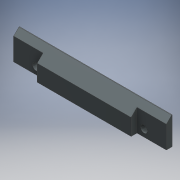
# Autodesk Inventor part: back_beam
Saved by Autodesk Inventor 2016 (Build 200138000, 138)
## iProperties
Created: 2017-01-15
Part Number: back_beam
Material: Generic
Document SubType Name: Modeling
Designer: hesaon
Density: 1 g/cm^3
Appearance: Default
Author: hesaon
Autodesk Inventor part; units mm, degrees
ref_plane "YZ Plane" through (0, 0, 0) normal (1, 0, 0) x (0, 1, 0)
ref_plane "XZ Plane" through (0, 0, 0) normal (0, 1, 0) x (-1, 0, 0)
ref_plane "XY Plane" through (0, 0, 0) normal (0, 0, 1) x (1, 0, 0)
sketch "Sketch1" plane through (0, 0, 0) normal (1, 0, 0) x (0, 1, 0)
  line L0 (0, 0) -> (0, -36)
  line L1 (0, -36) -> (-5, -36)
  line L2 (-5, -36) -> (-5, -5)
  line L3 (-5, -5) -> (0, 0)
  dimension "d1" = 5
  dimension "d2" = 45
  dimension "d5" = 31
  constraints: 8 end point, 2 perpendicular, 1 vertical
  measures "d1" distance of L0.end L1.end
  measures "d2" angle of L2 L3
  measures "d5" distance of L1.end L2.end
extrude "Extrusion1" add sketch "Sketch1" along normal blind 130
sketch "Sketch2" plane through (130, 0, 0) normal (1, 0, 0) x (0, 0, -1)
  line L0 (36, 0) -> (0, 0) projected
  line L1 (0, 0) -> (0.5, 0)
  line L2 (0.5, 0) -> (0.5, -0.5)
  line L3 (0, 0) -> (5, -5) projected
  line L4 (0, 0) -> (0.5, -0.5)
  dimension "d6" = 0.5
  constraints: 6 end point, 2 point on line, 1 collinear, 1 perpendicular
  measures "d6" distance of L0.end L1.end
extrude "Extrusion2" cut sketch "Sketch2" against normal through all
sketch "Sketch3" plane through (0, 0, -36) normal (0, 1, 0) x (1, 0, 0)
  circle A0 centre (19, -6) radius 3
  circle A1 centre (19, -18) radius 3
  line L0 (0, -35.5) -> (0, 0) projected
  line L1 (0, 0) -> (130, 0) projected
  circle A2 centre (111, -6) radius 3
  circle A3 centre (111, -18) radius 3
  line L2 (130, 0) -> (130, -35.5) projected
  point P0 (0, -36)
  dimension "d9" = 6
  dimension "d10" = 6
  dimension "d11" = 19
  dimension "d12" = 12
  dimension "d13" = 6
  dimension "d16" = 6
  dimension "d17" = 6
  dimension "d18" = 19
  dimension "d19" = 12
  constraints: 4 centre point, 2 vertical alignment, 1 horizontal alignment
  measures "d9" diameter of A0
  measures "d10" diameter of A1
  measures "d11" distance from line of L0 A0.centre
  measures "d12" distance of A1.centre A0.centre
  measures "d13" distance from line of L1 A0.centre
  measures "d16" diameter of A2
  measures "d17" diameter of A3
  measures "d18" distance from line of L2 A2.centre
  measures "d19" distance of A3.centre A2.centre
extrude "Extrusion4" cut sketch "Sketch3" against normal up to next
sketch "Sketch4" plane through (0, -5, -36) normal (0, -1, 0) x (1, 0, 0)
  line L0 (0, 0) -> (130, 0) projected
  line L1 (0, 31) -> (130, 31) projected
  line L2 (25, 0) -> (105, 0)
  line L3 (105, 0) -> (105, 31)
  line L4 (105, 31) -> (25, 31)
  line L5 (25, 31) -> (25, 0)
  line L6 (130, 31) -> (130, 0) projected
  point P0 (0, 36)
  dimension "d22" = 25
  dimension "d23" = 25
  constraints: 8 end point, 2 parallel, 2 point on line, 1 horizontal, 1 perpendicular
  measures "d22" distance between parallel lines of L6 L3
  measures "d23" distance of L0.start L2.start
extrude "Extrusion5" add sketch "Sketch4" along normal blind 5 contours L5 L1 L3 L0
sketch "Sketch5" plane through (25, -5, -36) normal (-1, 0, 0) x (0, 0, 1)
  line L0 (31, 0) -> (31, -5) projected
  line L1 (31, 0) -> (31, -5)
  line L2 (31, -5) -> (26, -5)
  line L3 (0, -5) -> (31, -5) projected
  line L4 (26, -5) -> (31, 0)
  point P0 (36, 5)
  dimension "d26" = 5
  constraints: 6 end point, 1 collinear, 1 point on line
  measures "d26" distance of L0.end L2.end
extrude "Extrusion6" cut sketch "Sketch5" against normal up to next
sketch "Sketch6" plane through (130, 0, 0) normal (1, 0, 0) x (0, 0, -1)
  line L0 (0.5, 0) -> (0.5, -0.5) projected
  line L1 (0.5, -0.5) -> (5, -5) projected
  line L2 (5, -5) -> (36, -5) projected
  line L3 (36, -5) -> (36, 0) projected
  line L4 (36, 0) -> (0.5, 0) projected
  line L5 (5, -5) -> (10, -10) projected
  line L6 (36, -10) -> (10, -10) projected
  line L7 (36, -5) -> (36, -10) projected
  line L8 (5, -5) -> (36, -5) projected
  line L9 (36, 0) -> (24, 0)
  line L10 (24, 0) -> (24, -5)
  line L11 (24, -5) -> (36, -5)
  line L12 (36, -5) -> (36, 0)
  point P0 (0, 0)
  dimension "d29" = 12
  dimension "d30" = 5
  constraints: 8 end point, 2 parallel, 1 horizontal, 1 perpendicular
  measures "d29" distance of L11.end L10.end
  measures "d30" distance of L10.end L9.end
extrude "Extrusion7" cut sketch "Sketch6" against normal through all contours L4 L3 L2 L10
sketch "Sketch7" plane through (105, -10, -10) normal (1, 0, 0) x (0, 0, -1)
  line L0 (-5, 5) -> (0, 0) projected
  line L1 (26, 0) -> (0, 0) projected
  line L2 (26, 5) -> (26, 0) projected
  line L3 (14, 5) -> (26, 5) projected
  line L4 (-5, 5) -> (14, 5) projected
  line L5 (14, 5) -> (14, 10) projected
  line L6 (14, 10) -> (-9.5, 10) projected
  line L7 (-9.5, 10) -> (-9.5, 9.5) projected
  line L8 (-9.5, 9.5) -> (-5, 5) projected
  line L9 (-5, 5) -> (14, 5) projected
  line L10 (26, 0) -> (14, 0)
  line L11 (14, 0) -> (14, 5)
  line L12 (14, 5) -> (26, 5)
  line L13 (26, 5) -> (26, 0)
  point P0 (-10, 10)
  constraints: 8 end point, 2 parallel, 1 horizontal, 1 perpendicular
extrude "Extrusion8" cut sketch "Sketch7" against normal through all contours L3 L2 L1 L11
body "Solid1"
